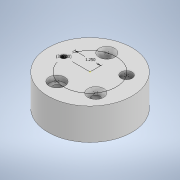
# Autodesk Inventor part: Hole Practice
Saved by Autodesk Inventor 2020 (Build 240168000, 168)
## iProperties
Created: 2020-01-30
Part Number: Hole Practice
Material: Generic
Document SubType Name: Modeling
Designer: cks4a449
Density: 1 g/cm^3
Appearance: Default
Author: cks4a449
Autodesk Inventor part; units mm, degrees
ref_plane "YZ Plane" through (0, 0, 0) normal (1, 0, 0) x (0, 1, 0)
ref_plane "XZ Plane" through (0, 0, 0) normal (0, 1, 0) x (-1, 0, 0)
ref_plane "XY Plane" through (0, 0, 0) normal (0, 0, 1) x (1, 0, 0)
sketch "Sketch1" plane through (0, 0, 0) normal (0, 1, 0) x (-1, 0, 0)
  circle A0 centre (0, 0) radius 50.8
  dimension "d0" = 101.6
  constraints: 1 centre point, 1 coincident
  measures "d0" diameter of A0
extrude "Extrusion1" add sketch "Sketch1" along normal blind 38.1
sketch "Sketch2" plane through (0, 38.1, 0) normal (0, 1, 0) x (1, 0, 0)
  point P0 (0, 0)
  point P1 (-31.75, 0)
  point P2 (-9.8113, -30.196)
  point P3 (25.6863, -18.6622)
  point P4 (25.6863, 18.6622)
  point P5 (-9.8113, 30.196)
  dimension "d3" = 31.75
  dimension "d4" = 0
  dimension "d7" = 360
  constraints: 6 other
  measures "d3" distance of point (0, 0) point (-31.75, 0)
  measures "d4" vertical distance of point (0, 0) point (-31.75, 0)
hole "Hole1" at (-31.75, 38.1, 0) direction (0, -1, 0) diameter 6.35 end through all
hole "Hole2" at (-9.8113, 38.1, 30.196) direction (0, -1, 0) diameter 9.525 end through all counterbore diameter 19.05 counterbore depth 6.35
hole "Hole3" at (25.6863, 38.1, 18.6622) direction (0, -1, 0) diameter 9.525 end through all countersink diameter 19.05 countersink angle 82
hole "Hole4" at (-9.8113, 38.1, -30.196) direction (0, -1, 0) diameter 4.9784 end through all countersink diameter 19.05 countersink angle 82 thread size "1/4-20 UNC" class "1B" standard "ANSI Unified Screw Threads"
hole "Hole5" at (25.6863, 38.1, -18.6622) direction (0, -1, 0) diameter 13.4874 end through all clearance for "Hex Head Bolt" size "1/2" standard "Ansi Unified Screw Threads"
body "Solid1"
